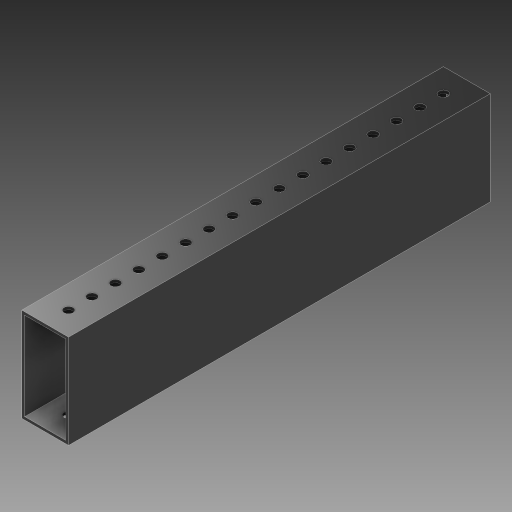
# Autodesk Inventor part: GreyT Claw 2 Main Tube 9 Gusset
Saved by Autodesk Inventor 2023 (Build 270158000, 158)
## iProperties
RuleStatus: InUse
Created: 2022-01-07
Part Number: GreyT Claw 2 Main Tube 9 Gusset
Material: Aluminum 6061
Document SubType Name: Modeling
Density: 2.7 g/cm^3
Appearance: Glossy - Black
Mass: 176.742 g
Surface Area: 844.055 cm^2
Volume: 65.46 cm^3
Autodesk Inventor part; units mm, degrees
ref_plane "YZ Plane" through (0, 0, 0) normal (1, 0, 0) x (0, 1, 0)
ref_plane "XZ Plane" through (0, 0, 0) normal (0, 1, 0) x (-1, 0, 0)
ref_plane "XY Plane" through (0, 0, 0) normal (0, 0, 1) x (1, 0, 0)
sketch "Sketch1" plane through (0, 0, 0) normal (0, 0, 1) x (1, 0, 0)
  line L0 (-12.7, -25.4) -> (12.7, -25.4)
  line L1 (12.7, -25.4) -> (12.7, 25.4)
  line L2 (12.7, 25.4) -> (-12.7, 25.4)
  line L3 (-12.7, 25.4) -> (-12.7, -25.4)
  line L4 (-12.7, -25.4) -> (12.7, 25.4) construction
  line L5 (12.7, -25.4) -> (-12.7, 25.4) construction
  line L6 (-11.1125, -23.8125) -> (11.1125, -23.8125)
  line L7 (11.1125, -23.8125) -> (11.1125, 23.8125)
  line L8 (11.1125, 23.8125) -> (-11.1125, 23.8125)
  line L9 (-11.1125, 23.8125) -> (-11.1125, -23.8125)
  point P0 (0, 0)
  dimension "d0" = 25.4
  dimension "d1" = 50.8
  dimension "d2" = 1.5875
  constraints: 20 end point, 4 parallel, 2 midpoint, 2 perpendicular, 1 horizontal, 3 other
  measures "d0" distance of L2.end L1.end
  measures "d1" distance of L1.end L0.end
  measures "d2" distance between parallel lines of L3 L9
extrude "BaseTube" add sketch "Sketch1" along normal mid plane 228.6
sketch "TopPoint" plane through (-12.7, 25.4, 114.3) normal (0, 1, 0) x (1, 0, 0)
  line L0 (25.4, 0) -> (0, 0) projected
  line L1 (0, 228.6) -> (0, 0) projected
  point P0 (12.7, 12.7)
  dimension "TLE_" = 12.7
  dimension "TWE_" = 12.7
  measures "TLE_" distance from line of L0 point (12.7, 12.7)
  measures "TWE_" distance from line of L1 point (12.7, 12.7)
sketch "SidePoint" plane through (12.7, -25.4, 114.3) normal (1, 0, 0) x (0, 0, -1)
  line L0 (0, 0) -> (0, 50.8) projected
  line L1 (228.6, 50.8) -> (0, 50.8) projected
  point P0 (88.9, 44.45)
  dimension "SLE_" = 88.9
  dimension "SWE_" = 6.35
  measures "SLE_" distance from line of point (88.9, 44.45) L0
  measures "SWE_" distance from line of point (88.9, 44.45) L1
hole "TopHole" at (0, 25.4, 101.6) direction (0, -1, 0) diameter 4.9784 end through all
hole "SideHole" [suppressed]
pattern_linear "TopPattern" count 9 spacing 12.7 along (0, 0, -1) of "TopHole"
pattern_linear "SidePattern" [suppressed]
mirror "TopMirror" about plane through (0, 0, 0) normal (0, 0, 1) of "TopHole", "TopPattern"
mirror "SideMirror" [suppressed]
sketch "Sketch4" plane through (-12.7, 25.4, 114.3) normal (0, 1, 0) x (1, 0, 0)
  line L0 (25.4, 228.6) -> (25.4, 0) projected
  line L1 (25.4, 0) -> (0, 0) projected
  line L2 (0, 228.6) -> (25.4, 228.6) projected
  line L3 (0, 228.6) -> (0, 0) projected
  line L4 (0, 0) -> (25.4, 25.4)
  line L5 (0, 228.6) -> (25.4, 203.2)
  dimension "d36" = 25.4
  constraints: 4 end point, 2 point on line, 1 perpendicular
  measures "d36" distance from line of L1 L4.end
extrude "CornerCut" [suppressed]
sketch "Sketch5" plane through (12.7, -25.4, 114.3) normal (1, 0, 0) x (0, 0, -1)
  circle A0 centre (31.75, 25.4) radius 14.2875
  line L0 (0, 0) -> (0, 50.8) projected
  point P0 (0, 25.4)
  dimension "d39" = 28.575
  dimension "d40" = 31.75
  constraints: 1 centre point, 1 horizontal alignment, 1 midpoint
  measures "d39" diameter of A0
  measures "d40" distance from line of A0.centre L0
extrude "FrontBearingHole" [suppressed]
sketch "Sketch6" plane through (12.7, -25.4, 114.3) normal (1, 0, 0) x (0, 0, -1)
  circle A0 centre (196.85, 25.4) radius 14.2875
  line L0 (228.6, 50.8) -> (228.6, 0) projected
  point P0 (228.6, 25.4)
  dimension "d43" = 28.575
  dimension "d44" = 31.75
  constraints: 1 centre point, 1 horizontal alignment, 1 midpoint
  measures "d43" diameter of A0
  measures "d44" distance from line of L0 A0.centre
extrude "BackBearingHole" [suppressed]
sketch "6wd" plane through (12.7, -25.4, 114.3) normal (1, 0, 0) x (0, 0, -1)
  circle A0 centre (-66.668, 25.4) radius 14.2875
  circle A1 centre (114.3, 23.8125) radius 14.2875
  circle A2 centre (295.268, 25.4) radius 14.2875
  line L0 (228.6, 50.8) -> (0, 50.8) projected
  line L1 (228.6, 0) -> (0, 0) construction
  arc A3 (-66.5085, 43.5907) -> (-66.8276, 7.2093) centre (-66.668, 25.4) ccw construction
  arc A4 (114.1404, 5.6218) -> (114.4596, 42.0032) centre (114.3, 23.8125) ccw construction
  line L2 (-66.5085, 43.5907) -> (114.4596, 42.0032) construction
  line L3 (114.1404, 5.6218) -> (-66.8276, 7.2093) construction
  circle A5 centre (-66.668, 25.4) radius 50.8 construction
  circle A6 centre (114.3, 23.8125) radius 50.8 construction
  circle A7 centre (295.268, 25.4) radius 50.8 construction
  point P0 (-49.8301, 8.562)
  point P1 (97.462, 40.6505)
  point P2 (278.4301, 42.238)
  point P3 (-42.8555, 25.4)
  point P4 (-49.8301, 42.238)
  point P5 (-66.668, 49.2125)
  point P6 (-83.506, 42.238)
  point P7 (-90.4805, 25.4)
  point P8 (-83.506, 8.562)
  point P9 (-66.668, 1.5875)
  point P10 (90.4875, 23.8125)
  point P11 (97.462, 6.9745)
  point P12 (114.3, 0)
  point P13 (131.138, 6.9745)
  point P14 (138.1125, 23.8125)
  point P15 (131.138, 40.6505)
  point P16 (114.3, 47.625)
  point P17 (271.4555, 25.4)
  point P18 (278.4301, 8.562)
  point P19 (295.268, 1.5875)
  point P20 (312.106, 8.562)
  point P21 (319.0805, 25.4)
  point P22 (312.106, 42.238)
  point P23 (295.268, 49.2125)
  point P24 (114.3, 50.8)
  point P25 (-123.818, 25.4)
  point P26 (57.15, 23.8125)
  point P27 (238.118, 25.4)
  point P28 (-9.518, 25.4)
  point P29 (171.45, 23.8125)
  point P30 (352.418, 25.4)
  point P31 (-28.568, 26.9875)
  point P32 (257.168, 26.9875)
  point P33 (152.4, 26.9875)
  point P34 (76.2, 26.9875)
  dimension "d47" = 28.575
  dimension "d50" = 315
  dimension "d52" = 25.4
  dimension "d55" = 315
  dimension "d59" = 315
  dimension "d61" = 23.8125
  dimension "d62" = 23.8125
  dimension "d63" = 23.8125
  dimension "d64" = 26.9875
  dimension "d68" = 36.3828
  dimension "d69" = 57.15
  dimension "d70" = 180.975
  dimension "d71" = 57.15
  dimension "d72" = 180.975
  dimension "d73" = 180.975
  dimension "d74" = 101.6
  dimension "d131" = 180
  dimension "d133" = 114.3
  dimension "d136" = 360
  dimension "d140" = 360
  dimension "d142" = 114.3
  dimension "d143" = 114.3
  dimension "d186" = 38.1
  dimension "d187" = 38.1
  dimension "d188" = 38.1
  dimension "d189" = 38.1
  dimension "d190" = 23.8125
  constraints: 8 centre point, 8 horizontal alignment, 5 coincident, 5 equal radius, 4 end point, 4 point on circle, 4 tangent, 3 vertical alignment, 1 midpoint, 38 other
  measures "d47" diameter of A0
  measures "d52" distance from line of A0.centre L0
  measures "d61" distance of A0.centre point (-66.668, 1.588)
  measures "d62" distance of point (114.3, 47.625) A1.centre
  measures "d63" distance of point (295.268, 49.212) A2.centre
  measures "d64" distance from line of A1.centre L0
  measures "d68" diameter of A3
  measures "d70" distance of L3.start L3.end
  measures "d72" distance of L2.start L2.end
  measures "d73" distance of A2.centre A1.centre
  measures "d74" diameter of A5
  measures "d133" distance of point (-9.518, 25.4) point (-123.818, 25.4)
  measures "d142" distance of point (171.45, 23.812) point (57.15, 23.812)
  measures "d143" distance of point (352.418, 25.4) point (238.118, 25.4)
  measures "d186" horizontal distance of A0.centre point (-28.568, 26.988)
  measures "d187" horizontal distance of point (257.168, 26.988) A2.centre
  measures "d188" horizontal distance of A1.centre point (76.2, 26.988)
  measures "d189" horizontal distance of point (152.4, 26.988) A1.centre
  measures "d190" distance from line of L0 point (-28.568, 26.988)
extrude "6wdBearings" [suppressed]
hole "6wdBearingBlocks" [suppressed]
sketch "8wd" plane through (12.7, -25.4, 114.3) normal (1, 0, 0) x (0, 0, -1)
  circle A0 centre (-71.3968, 26.9875) radius 14.2875
  circle A1 centre (52.3875, 23.8125) radius 14.2875
  circle A2 centre (176.2125, 23.8125) radius 14.2875
  circle A3 centre (299.9968, 26.9875) radius 14.2875
  line L0 (228.6, 50.8) -> (0, 50.8) projected
  arc A4 (-70.9303, 45.1729) -> (-71.8632, 8.8021) centre (-71.3968, 26.9875) ccw construction
  arc A5 (51.9211, 5.6271) -> (52.8539, 41.9979) centre (52.3875, 23.8125) ccw construction
  line L1 (-70.9303, 45.1729) -> (52.8539, 41.9979) construction
  line L2 (51.9211, 5.6271) -> (-71.8632, 8.8021) construction
  arc A6 (176.2125, 5.6211) -> (176.2125, 42.0039) centre (176.2125, 23.8125) ccw construction
  arc A7 (52.3875, 42.0039) -> (52.3875, 5.6211) centre (52.3875, 23.8125) ccw construction
  line L3 (52.3875, 42.0039) -> (176.2125, 42.0039) construction
  line L4 (52.3875, 5.6211) -> (176.2125, 5.6211) construction
  line L5 (114.3, 50.8) -> (114.3, 0) construction
  line L6 (0, 0) -> (228.6, 0) projected
  circle A8 centre (-71.3968, 26.9875) radius 50.8 construction
  circle A9 centre (52.3875, 23.8125) radius 50.8 construction
  circle A10 centre (176.2125, 23.8125) radius 50.8 construction
  circle A11 centre (299.9968, 26.9875) radius 50.8 construction
  line L7 (0, 0) -> (0, 50.8) projected
  line L8 (228.6, 50.8) -> (228.6, 0) projected
  point P0 (-71.3968, 50.8)
  point P1 (52.3875, 47.625)
  point P2 (176.2125, 47.625)
  point P3 (299.9968, 50.8)
  point P4 (-88.2348, 43.8255)
  point P5 (-95.2093, 26.9875)
  point P6 (-88.2348, 10.1495)
  point P7 (-71.3968, 3.175)
  point P8 (-54.5588, 10.1495)
  point P9 (-47.5843, 26.9875)
  point P10 (-54.5588, 43.8255)
  point P11 (35.5495, 40.6505)
  point P12 (28.575, 23.8125)
  point P13 (35.5495, 6.9745)
  point P14 (52.3875, 0)
  point P15 (69.2255, 6.9745)
  point P16 (76.2, 23.8125)
  point P17 (69.2255, 40.6505)
  point P18 (159.3745, 40.6505)
  point P19 (152.4, 23.8125)
  point P20 (159.3745, 6.9745)
  point P21 (176.2125, 0)
  point P22 (193.0505, 6.9745)
  point P23 (200.025, 23.8125)
  point P24 (193.0505, 40.6505)
  point P25 (283.1588, 43.8255)
  point P26 (276.1843, 26.9875)
  point P27 (283.1588, 10.1495)
  point P28 (299.9968, 3.175)
  point P29 (316.8348, 10.1495)
  point P30 (323.8093, 26.9875)
  point P31 (316.8348, 43.8255)
  point P32 (-128.5468, 26.9875)
  point P33 (-14.2468, 26.9875)
  point P34 (-4.7625, 23.8125)
  point P35 (119.0625, 23.8125)
  point P36 (242.8468, 26.9875)
  point P37 (109.5375, 23.8125)
  point P38 (233.3625, 23.8125)
  point P39 (357.1468, 26.9875)
  point P40 (-33.3299, 25.4)
  point P41 (14.2875, 25.4)
  point P42 (90.4875, 25.4)
  point P43 (138.1125, 25.4)
  point P44 (214.3125, 25.4)
  point P45 (261.9299, 25.4)
  dimension "d84" = 28.575
  dimension "d86" = 26.9875
  dimension "d87" = 23.8125
  dimension "d88" = 23.8125
  dimension "d89" = 23.8125
  dimension "d90" = 23.8125
  dimension "d93" = 360
  dimension "d97" = 360
  dimension "d101" = 360
  dimension "d105" = 360
  dimension "d107" = 36.3828
  dimension "d108" = 57.15
  dimension "d109" = 123.825
  dimension "d110" = 57.15
  dimension "d111" = 123.825
  dimension "d112" = 123.825
  dimension "d113" = 36.3828
  dimension "d114" = 57.15
  dimension "d115" = 123.825
  dimension "d116" = 57.15
  dimension "d117" = 123.825
  dimension "d118" = 61.9125
  dimension "d119" = 101.6
  dimension "d206" = 23.8125
  dimension "d211" = 360
  dimension "d213" = 114.3
  dimension "d216" = 360
  dimension "d218" = 114.3
  dimension "d221" = 360
  dimension "d223" = 114.3
  dimension "d226" = 360
  dimension "d228" = 114.3
  dimension "d285" = 25.4
  dimension "d286" = 38.1
  dimension "d287" = 38.1
  dimension "d288" = 38.1
  dimension "d289" = 38.1
  dimension "d290" = 38.1
  dimension "d291" = 38.1
  constraints: 12 centre point, 12 end point, 11 horizontal alignment, 8 coincident, 8 equal radius, 8 point on circle, 6 tangent, 4 vertical alignment, 2 midpoint, 1 parallel, 48 other
  measures "d84" diameter of A0
  measures "d86" distance from line of A1.centre L0
  measures "d87" distance of point (-71.397, 50.8) A0.centre
  measures "d88" distance of A1.centre point (52.387, 47.625)
  measures "d89" distance of A2.centre point (176.213, 47.625)
  measures "d90" distance of A3.centre point (299.997, 50.8)
  measures "d107" diameter of A4
  measures "d109" distance of L2.start L2.end
  measures "d111" distance of L1.start L1.end
  measures "d112" distance of A3.centre A2.centre
  measures "d113" diameter of A6
  measures "d115" distance of L4.start L4.end
  measures "d117" distance of L3.start L3.end
  measures "d118" distance from line of A1.centre L5
  measures "d119" diameter of A8
  measures "d206" distance from line of A0.centre L0
  measures "d213" distance of point (-14.247, 26.988) point (-128.547, 26.988)
  measures "d218" distance of point (109.537, 23.812) point (-4.763, 23.812)
  measures "d223" distance of point (233.363, 23.812) point (119.062, 23.812)
  measures "d228" distance of point (357.147, 26.987) point (242.847, 26.987)
  measures "d285" distance from line of point (-33.33, 25.4) L0
  measures "d286" distance of A0.centre point (-33.33, 25.4)
  measures "d287" horizontal distance of A1.centre point (14.287, 25.4)
  measures "d288" horizontal distance of point (90.487, 25.4) A1.centre
  measures "d289" horizontal distance of A2.centre point (138.112, 25.4)
  measures "d290" horizontal distance of point (214.312, 25.4) A2.centre
  measures "d291" distance of A3.centre point (261.93, 25.4)
extrude "8wdBearings" [suppressed]
hole "8wdBearingBlocks" [suppressed]
sketch "6wdPoints" plane through (-12.7, -25.4, 114.3) normal (-1, 0, 0) x (0, 0, 1)
  point P0 (123.818, 25.4)
  point P1 (9.518, 25.4)
  point P2 (-57.15, 23.8125)
  point P3 (-171.45, 23.8125)
  point P4 (-238.118, 25.4)
  point P5 (-352.418, 25.4)
  point P6 (28.568, 26.9875)
  point P7 (-76.2, 26.9875)
  point P8 (-152.4, 26.9875)
  point P9 (-257.168, 26.9875)
hole "FL6wdGB" [suppressed]
hole "ML6wdGB" [suppressed]
hole "BL6wdGB" [suppressed]
hole "FR6wdGB" [suppressed]
hole "MR6wdGB" [suppressed]
hole "BR6wdGB" [suppressed]
hole "CL6wd" [suppressed]
hole "CR6wd" [suppressed]
sketch "Sketch10" plane through (-12.7, -25.4, 114.3) normal (-1, 0, 0) x (0, 0, 1)
  point P0 (128.5468, 26.9875)
  point P1 (14.2468, 26.9875)
  point P2 (4.7625, 23.8125)
  point P3 (-109.5375, 23.8125)
  point P4 (-119.0625, 23.8125)
  point P5 (-233.3625, 23.8125)
  point P6 (-242.8468, 26.9875)
  point P7 (-357.1468, 26.9875)
hole "FL8wdGB" [suppressed]
hole "FMdL8wdGB" [suppressed]
hole "BMdL8wdGB" [suppressed]
hole "BL8wdGB" [suppressed]
hole "FR8wdGB" [suppressed]
hole "FMdR8wdGB" [suppressed]
hole "BMdR8wdGB" [suppressed]
hole "BR8wdGB" [suppressed]
hole "CL8wd" [suppressed]
sketch "Sketch11" plane through (-12.7, -25.4, 114.3) normal (-1, 0, 0) x (0, 0, 1)
  line L0 (-228.6, 50.8) -> (0, 50.8) projected
  line L1 (0, 0) -> (0, 50.8) projected
  line L2 (0, 0) -> (-228.6, 0) projected
  line L3 (-228.6, 50.8) -> (-228.6, 0) projected
  point P0 (33.3299, 25.4)
  point P1 (-14.2875, 25.4)
  point P2 (-90.4875, 25.4)
  point P3 (-138.1125, 25.4)
  point P4 (-214.3125, 25.4)
  point P5 (-261.9299, 25.4)
hole "CR8wd" [suppressed]
sketch "Sketch12" plane through (-12.7, -25.4, 114.3) normal (-1, 0, 0) x (0, 0, 1)
  circle A0 centre (-152.4, 44.45) radius 2.4892 projected
  circle A1 centre (-152.4, 31.75) radius 2.4892 projected
  circle A2 centre (-152.4, 19.05) radius 2.4892 projected
  circle A3 centre (-152.4, 6.35) radius 2.4892 projected
  circle A4 centre (-88.9, 44.45) radius 2.4892 projected
  circle A5 centre (-88.9, 31.75) radius 2.4892 projected
  circle A6 centre (-88.9, 19.05) radius 2.4892 projected
  circle A7 centre (-88.9, 6.35) radius 2.4892 projected
  point P0 (-88.9, 31.75)
  constraints: 8 coincident
hole "Hole23" [suppressed]
equation "\"d0\" = Width"
equation "\"d1\" = Height"
equation "\"d2\" = Wall"
equation "\"d3\" = Length"
equation "\"d62\" = d61"
equation "\"d63\" = d61"
equation "\"d6\" = HoleSize"
equation "\"d73\" = d72"
equation "\"d77\" = HoleSize"
equation "\"Height\" = 50.8"
equation "\"Width\" = 25.4"
equation "\"Wall\" = 1.5875"
equation "\"Length\" = 228.6"
equation "\"Top_Lengthwise_Space\" = 12.7"
equation "\"Top_Widthwise_Space\" = 12.7"
equation "\"Top_Lengthwise_Edge\" = 12.7"
equation "\"Top_Widthwise_Edge\" = 12.7"
equation "\"Side_Lengthwise_Edge\" = 88.9"
equation "\"Side_Widthwise_Edge\" = 12.7"
equation "\"Side_Lengthwise_Space\" = 12.7"
equation "\"Side_Widthwise_Space\" = 12.7"
equation "\"HoleSize\" = 4.9784"
body "Solid1"
